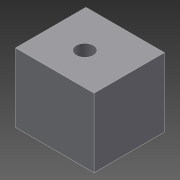
# Autodesk Inventor part: REBASE_TEST
Saved by Autodesk Inventor 2014 SP1 (Build 180222100, 222)
## iProperties
Created: 2014-03-23
Part Number: REBASE_TEST
Material: Generic
Document SubType Name: Modeling
Designer: Mark
Density: 1 g/cm^3
Appearance: Default
Author: Mark
Autodesk Inventor part; units mm, degrees
ref_plane "Right (YZ)" through (0, 0, 0) normal (1, 0, 0) x (0, 1, 0)
ref_plane "Top (XZ)" through (0, 0, 0) normal (0, 1, 0) x (-1, 0, 0)
ref_plane "Front (XY)" through (0, 0, 0) normal (0, 0, 1) x (1, 0, 0)
sketch "Sketch1" plane through (0, 0, 0) normal (0, 1, 0) x (-1, 0, 0)
  line L0 (-14.4744, -12.9757) -> (14.4744, -12.9757)
  line L1 (14.4744, -12.9757) -> (14.4744, 12.9757)
  line L2 (14.4744, 12.9757) -> (-14.4744, 12.9757)
  line L3 (-14.4744, 12.9757) -> (-14.4744, -12.9757)
  line L4 (-14.4744, -12.9757) -> (14.4744, 12.9757) construction
  line L5 (14.4744, -12.9757) -> (-14.4744, 12.9757) construction
  point P0 (0, 0)
  constraints: 12 end point, 2 midpoint, 2 parallel, 1 horizontal, 1 perpendicular
extrude "Extrusion1" add sketch "Sketch1" along normal blind 25.4
hole "Hole1" at (-0.9144, 25.4, 0.9803) direction (0, -1, 0) diameter 6.35 end through all
body "Solid1"
